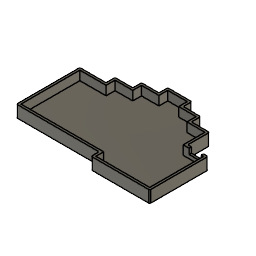
right_bottom (Autodesk Fusion 360 design; units mm, degrees)
part number: 2026-06-19-20-55-49-517
Autodesk Fusion 360 part; units mm, degrees
note: some values were not read from the file. Set by a fixed rule: which sketch regions a step uses.
sketch "Sketch2" plane through (0, 0, 0) normal (0, 0, 1) x (1, 0, 0)
  line L0 (67.3808, -47.0282) -> (8.2999, -46.9982)
  line L1 (-53.4602, 26) -> (-53.4553, 35.7749)
  line L2 (-14.8719, 54.9669) -> (6.5299, 54.9669)
  line L3 (-82.208, 26) -> (-53.4602, 26)
  line L4 (8.2999, -46.9982) -> (8.3043, -38.4744)
  line L5 (-14.8719, 45.3124) -> (-14.8719, 54.9669)
  line L6 (-33.9828, 35.7749) -> (-33.9779, 45.3221)
  line L7 (6.5299, 45.6019) -> (25.5899, 45.5869)
  line L8 (-33.9779, 45.3221) -> (-14.8719, 45.3124)
  line L9 (45.2699, 35.5117) -> (45.2899, 11.7819)
  line L10 (25.5899, 35.5117) -> (45.2699, 35.5117)
  line L11 (45.2899, 11.7819) -> (67.3808, 11.8005)
  line L12 (6.5299, 54.9669) -> (6.5299, 45.6019)
  line L13 (8.3043, -38.4744) -> (-82.2408, -38.4911)
  line L14 (25.5899, 45.5869) -> (25.5899, 35.5606)
  line L15 (-53.4553, 35.7749) -> (-33.9828, 35.7749)
  line L16 (25.5899, 35.5606) -> (25.5899, 35.5117)
  line L17 (67.3808, 11.8005) -> (67.3808, -47.0282)
  line L18 (-82.2408, -38.4911) -> (-82.208, 26)
  line L19 (-55.9553, 28.5) -> (-84.708, 28.5)
  line L20 (-55.9553, 38.2749) -> (-55.9553, 28.5)
  line L21 (-55.9553, 38.2749) -> (-36.4828, 38.2749)
  line L22 (-36.4828, 38.2749) -> (-36.4828, 47.8221)
  line L23 (-36.4828, 47.8221) -> (-17.3719, 47.8221)
  line L24 (-17.3719, 47.8221) -> (-17.3719, 57.4669)
  line L25 (-17.3719, 57.4669) -> (9.0299, 57.4669)
  line L26 (9.0299, 57.4669) -> (9.0299, 48.0869)
  line L27 (28.0899, 48.0869) -> (9.0299, 48.0869)
  line L28 (28.0899, 48.0869) -> (28.0899, 38.0117)
  line L29 (28.0899, 38.0117) -> (47.7699, 38.0117)
  line L30 (47.7699, 38.0117) -> (47.7699, 14.3005)
  line L31 (69.8808, 14.3005) -> (47.7699, 14.3005)
  line L32 (69.8808, 14.3005) -> (69.8808, -49.5282)
  line L33 (69.8808, -49.5282) -> (5.7999, -49.5282)
  line L34 (5.7999, -49.5282) -> (5.7999, -40.9744)
  line L35 (5.7999, -40.9744) -> (-84.708, -40.9744)
  line L36 (-84.708, -40.9744) -> (-84.708, 28.5)
  dimension "d20" = 2.5
  dimension "d21" = 2.5
  dimension "d22" = 2.5
  dimension "d23" = 2.5
  dimension "d26" = 2.5
  dimension "d27" = 2.5
  dimension "d28" = 2.5
  dimension "d29" = 2.5
  dimension "d30" = 2.5
  dimension "d31" = 2.5
  dimension "d32" = 2.5
  dimension "d35" = 2.5
  dimension "d36" = 2.5
  dimension "d38" = 2.5
  dimension "d39" = 2.5
  dimension "d40" = 2.5
  dimension "d41" = 2.5
  dimension "d42" = 2.5
  dimension "d43" = 2.5
  constraint parallel L1 L18
  constraint parallel L3 L15
  constraint parallel L6 L18
  constraint perpendicular L6 L8
  constraint vertical L5
  constraint perpendicular L2 L5
  constraint perpendicular L2 L12
  constraint parallel L12 L14
  constraint perpendicular L7 L16
  constraint perpendicular L10 L12
  constraint perpendicular L9 L11
  constraint perpendicular L10 L17
  constraint perpendicular L0 L4
  constraint horizontal L19
  constraint vertical L20
  constraint horizontal L21
  constraint perpendicular L21 L22
  constraint perpendicular L5 L23
  constraint perpendicular L23 L24
  constraint coincident L23 L24.start
  constraint horizontal L25
  constraint coincident L24.end L25
  constraint vertical L26
  constraint perpendicular L26 L27
  constraint coincident L26 L27.end
  constraint vertical L28
  constraint coincident L27.start L28
  constraint horizontal L29
  constraint perpendicular L29 L30
  constraint horizontal L31
  constraint perpendicular L31 L32
  constraint perpendicular L17 L33
  constraint coincident L32 L33.start
  constraint perpendicular L33 L34
  constraint coincident L33.end L34
  constraint horizontal L35
  constraint coincident L34.end L35
  constraint perpendicular L35 L36
  constraint coincident L19.end L36
  constraint coincident L35 L36.start
  measures "d20" vertical distance of L3.start L19.end
  measures "d21" horizontal distance of L1.end L20.start
  measures "d22" vertical distance of L1.start L19.start
  measures "d23" vertical distance of L1.end L20.start
  measures "d26" horizontal distance of L6.start L21.end
  measures "d27" vertical distance of L6.end L22.end
  measures "d28" horizontal distance of L2.start L24.end
  measures "d29" vertical distance of L2.start L24.end
  measures "d30" horizontal distance of L2.end L25.end
  measures "d31" vertical distance of L7.end L27.start
  measures "d32" horizontal distance of L7.end L27.start
  measures "d35" vertical distance of L9.start L29.end
  measures "d36" horizontal distance of L9.start L29.end
  measures "d38" vertical distance of L11.end L30.end
  measures "d39" horizontal distance of L11.end L31.start
  measures "d40" vertical distance of L0.start L32.end
  measures "d41" horizontal distance of L0.end L33.end
  measures "d42" vertical distance of L4.end L34.end
  measures "d43" horizontal distance of L3.start L19.end
extrude "Extrude1" add sketch "Sketch2" along normal blind 3 contours L0 L1 L2 L3 L4 L5 L6 L7 L8 L9 L10 L11 L12 L13 L14 L15 L16 L17 L18
extrude "Extrude2" add sketch "Sketch2" along normal blind 13
sketch "Sketch3" plane through (0, 0, 13) normal (0, 0, 1) x (-1, 0, 0)
  line L0 (-8.3043, 38.4744) -> (82.2408, 38.4911)
  line L1 (82.2408, 38.4911) -> (82.208, -26)
  line L2 (82.208, -26) -> (53.4602, -26)
  line L3 (53.4602, -26) -> (53.4553, -35.7749)
  line L4 (53.4553, -35.7749) -> (33.9828, -35.7749)
  line L5 (33.9828, -35.7749) -> (33.9779, -45.3221)
  line L6 (33.9779, -45.3221) -> (14.8719, -45.3124)
  line L7 (14.8719, -45.3124) -> (14.8719, -54.9669)
  line L8 (14.8719, -54.9669) -> (-6.5299, -54.9669)
  line L9 (-6.5299, -54.9669) -> (-6.5299, -45.6019)
  line L10 (-6.5299, -45.6019) -> (-25.5899, -45.5869)
  line L11 (-25.5899, -45.5869) -> (-25.5899, -35.5606)
  line L12 (-25.5899, -35.5606) -> (-25.5899, -35.5117)
  line L13 (-25.5899, -35.5117) -> (-45.2699, -35.5117)
  line L14 (-45.2699, -35.5117) -> (-45.2899, -11.7819)
  line L15 (-45.2899, -11.7819) -> (-67.3808, -11.8005)
  line L16 (-67.3808, -11.8005) -> (-67.3808, 47.0282)
  line L17 (-67.3808, 47.0282) -> (-8.2999, 46.9982)
  line L18 (-8.2999, 46.9982) -> (-8.3043, 38.4744)
  line L19 (-69.8808, -14.3005) -> (-47.7699, -14.3005)
  line L20 (-47.7699, -14.3005) -> (-47.7699, -38.0117)
  line L21 (-47.7699, -38.0117) -> (-28.0899, -38.0117)
  line L22 (-28.0899, -38.0117) -> (-28.0899, -48.0869)
  line L23 (-28.0899, -48.0869) -> (-9.0299, -48.0869)
  line L24 (-9.0299, -48.0869) -> (-9.0299, -57.4669)
  line L25 (-9.0299, -57.4669) -> (17.3719, -57.4669)
  line L26 (17.3719, -57.4669) -> (17.3719, -47.8221)
  line L27 (17.3719, -47.8221) -> (36.4828, -47.8221)
  line L28 (36.4828, -47.8221) -> (36.4828, -38.2749)
  line L29 (36.4828, -38.2749) -> (55.9553, -38.2749)
  line L30 (55.9553, -38.2749) -> (55.9553, -28.5)
  line L31 (55.9553, -28.5) -> (84.708, -28.5)
  line L32 (84.708, -28.5) -> (84.708, 40.9744)
  line L33 (84.708, 40.9744) -> (-5.7999, 40.9744)
  line L34 (-5.7999, 40.9744) -> (-5.7999, 49.5282)
  line L35 (-5.7999, 49.5282) -> (-69.8808, 49.5282)
  line L36 (-69.8808, 49.5282) -> (-69.8808, -14.3005)
  line L37 (-51.7808, -15.1939) -> (-64.7808, -15.1939)
  line L38 (-64.7808, -15.1939) -> (-64.7808, -11.2822)
  line L39 (-64.7808, -11.2822) -> (-51.7808, -11.2822)
  line L40 (-51.7808, -11.2822) -> (-51.7808, -15.1939)
  dimension "d48" = 13
  dimension "d49" = 5.1
  constraint horizontal L37
  constraint vertical L38
  constraint horizontal L39
  constraint vertical L40
  measures "d48" distance of L38 L40
  measures "d49" horizontal distance of L19.start L38.end
extrude "Extrude3" cut sketch "Sketch3" against normal blind 6 contours L15 L19 L38 L40
fillet "Fillet1" radius 1 18 edges at (5.7999, -49.5282, 6.5) (-84.708, -40.9744, 6.5) (69.8808, -49.5282, 6.5) (5.7999, -40.9744, 6.5) (-84.708, 28.5, 6.5) (-55.9553, 38.2749, 6.5) (-36.4828, 47.8221, 6.5) (-17.3719, 57.4669, 6.5) (-55.9553, 28.5, 6.5) (-36.4828, 38.2749, 6.5) (-17.3719, 47.8221, 6.5) (28.0899, 48.0869, 6.5) (9.0299, 57.4669, 6.5) (47.7699, 38.0117, 6.5) (69.8808, 14.3005, 6.5) (28.0899, 38.0117, 6.5) (9.0299, 48.0869, 6.5) (47.7699, 14.3005, 6.5)
